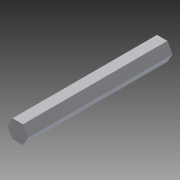
# Autodesk Inventor part: Hex Shaft Aluminum 1-2 in (am-2291)
Saved by Autodesk Inventor 2014 (Build 180170000, 170)
## iProperties
Created: 2014-01-12
Part Number: Hex Shaft Aluminum 1-2 in (am-2291)
Material: Aluminum 6061
Document SubType Name: Modeling
Designer: Michael
Density: 2.71 g/cm^3
Appearance: Aluminum - Flat
Author: Michael
Autodesk Inventor part; units mm, degrees
ref_plane "YZ Plane" through (0, 0, 0) normal (1, 0, 0) x (0, 1, 0)
ref_plane "XZ Plane" through (0, 0, 0) normal (0, 1, 0) x (-1, 0, 0)
ref_plane "XY Plane" through (0, 0, 0) normal (0, 0, 1) x (1, 0, 0)
sketch "Sketch1" plane through (0, 0, 0) normal (0, 0, 1) x (1, 0, 0)
  line L0 (3.6662, 6.35) -> (7.3323, 0)
  line L1 (7.3323, 0) -> (3.6662, -6.35)
  line L2 (3.6662, -6.35) -> (-3.6662, -6.35)
  line L3 (-3.6662, -6.35) -> (-7.3323, 0)
  line L4 (-7.3323, 0) -> (-3.6662, 6.35)
  line L5 (-3.6662, 6.35) -> (3.6662, 6.35)
  point P0 (0, 0)
  point P1 (0, 0)
  dimension "d0" = 12.7
  constraints: 12 end point, 1 coincident, 1 horizontal, 13 other
  measures "d0" distance between parallel lines of L2 L5
extrude "Extrusion1" add sketch "Sketch1" along normal blind 101.6
body "Solid1"
